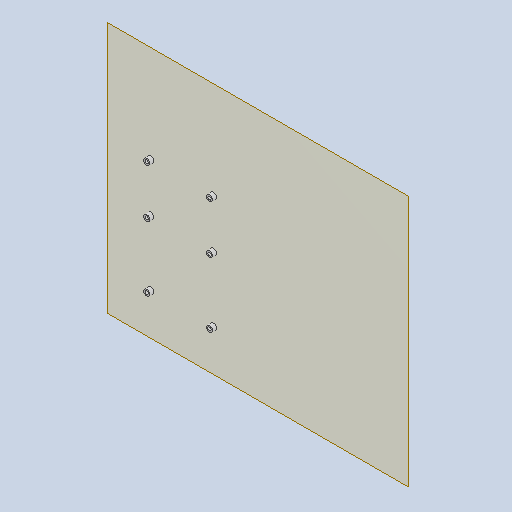
# Autodesk Inventor part: проставка платы
Saved by Autodesk Inventor 2024.2 (Build 282272000, 272)
## iProperties
Created: 2025-12-10
Part Number: проставка платы
Material: Типовые
Document SubType Name: Modeling
Designer: katya_notebook
Density: 1 g/cm^3
Appearance: По умолчанию
Author: katya_notebook
Autodesk Inventor part; units mm, degrees
ref_plane "YZ Plane" through (0, 0, 0) normal (1, 0, 0) x (0, 1, 0)
ref_plane "XZ Plane" through (0, 0, 0) normal (0, 1, 0) x (-1, 0, 0)
ref_plane "XY Plane" through (0, 0, 0) normal (0, 0, 1) x (1, 0, 0)
ref_plane "РабПлоскость1" through (216.9124, 167.0229, 0) normal (0, 0, 1) x (-1, -0.0002, 0)
sketch "Эскиз1" plane through (216.9124, 167.0229, 0) normal (0, 0, 1) x (-1, -0.0002, 0)
  circle A0 centre (106, 83.5) radius 1.6 projected
  circle A1 centre (44, 83.5) radius 1.6 projected
  circle A2 centre (44, 19.5) radius 1.6 projected
  circle A3 centre (106, 19.5) radius 1.6 projected
  circle A4 centre (106, -28.5) radius 1.6 projected
  circle A5 centre (44, -28.5) radius 1.6 projected
  circle A6 centre (106, -28.5) radius 3
  circle A7 centre (44, -28.5) radius 3
  circle A8 centre (106, 19.5) radius 3
  circle A9 centre (44, 19.5) radius 3
  circle A10 centre (44, 83.5) radius 3
  circle A11 centre (106, 83.5) radius 3
  point P0 (216.9474, 166.9774)
  dimension "d0" = 6
  dimension "d1" = 6
  constraints: 6 centre point, 6 coincident
  measures "d0" diameter of A6
  measures "d1" diameter of A7
extrude "Выдавливание1" add sketch "Эскиз1" along normal blind 4
